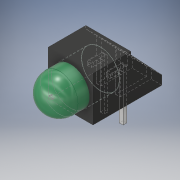
# Autodesk Inventor part: L-1503CB 1GD
Saved by Autodesk Inventor 2019.1 (Build 231200000, 200)
## iProperties
Created: 2021-06-01
Part Number: L-1503CB 1GD
Material: Типовые
Document SubType Name: Modeling
Designer: shawn
Density: 1 g/cm^3
Appearance: По умолчанию
Author: shawn
Autodesk Inventor part; units mm, degrees
ref_plane "YZ Plane" through (0, 0, 0) normal (1, 0, 0) x (0, 1, 0)
ref_plane "XZ Plane" through (0, 0, 0) normal (0, 1, 0) x (-1, 0, 0)
sketch "Эскиз1" plane through (0, 0, 0) normal (1, 0, 0) x (0, 1, 0)
  line L0 (0, 0) -> (6, 0)
  line L1 (6, 0) -> (6, -5.0448)
  line L2 (1.2044, -9.2) -> (0, -9.2)
  line L3 (0, -9.2) -> (0, 0)
  line L4 (1.2044, -9.2) -> (5.6, -5.0448)
  line L5 (5.6, -5.0448) -> (6, -5.0448)
  line L6 (11.4478, 9.2277) -> (11.4478, -15.7017) construction
  line L7 (11.4478, -15.7017) -> (-10.569, -15.7017) construction
  line L8 (-10.569, -15.7017) -> (-10.569, 9.2277) construction
  line L9 (-10.569, 9.2277) -> (11.4478, 9.2277) construction
  dimension "d2" = 0.4
  dimension "d39" = 6
  dimension "d40" = 9.2
  constraints: 13 end point, 2 parallel, 2 perpendicular, 1 horizontal, 3 other
  measures "d2" distance of L1.end L4.end
  measures "d39" distance of L0.start L0.end
  measures "d40" distance of L2.end L0.start
extrude "Выдавливание1" add sketch "Эскиз1" along normal mid plane 6
sketch "Эскиз2" plane through (-3, 0, 0) normal (0, 0, 1) x (1, 0, 0)
  line L0 (6, 6) -> (6, 0) construction
  line L1 (0, 0) -> (6, 6) construction
  line L2 (0, 0) -> (6, 0) construction
  line L3 (6, 0) -> (0, 6) construction
  line L4 (6, 6) -> (0, 6) construction
  circle A0 centre (3, 3) radius 2.55
  point P0 (3, 0)
  dimension "d43" = 5.1
  constraints: 5 end point, 1 centre point, 1 midpoint, 1 perpendicular
  measures "d43" diameter of A0
extrude "Выдавливание2" cut sketch "Эскиз2" against normal blind 4
sketch "Эскиз3" plane through (-3, 0, -9.2) normal (0, -1, 0) x (1, 0, 0)
  line L0 (6, 4.1552) -> (0, 4.1552) construction
  line L1 (6, 0) -> (0, 0) projected
  line L2 (4.57, 4.1552) -> (3.97, 4.1552)
  line L3 (3.97, 4.1552) -> (3.97, 0)
  line L4 (3.97, 0) -> (4.57, 0)
  line L5 (4.57, 0) -> (4.57, 4.1552)
  line L6 (6, 4.1552) -> (0, 4.1552) construction
  line L7 (3, 4.1552) -> (3, 0) construction
  line L8 (1.43, 4.1552) -> (2.03, 4.1552)
  line L9 (2.03, 4.1552) -> (2.03, 0)
  line L10 (2.03, 0) -> (1.43, 0)
  line L11 (1.43, 0) -> (1.43, 4.1552)
  point P0 (3, 9.2)
  point P1 (4.27, 0)
  point P2 (1.73, 0)
  dimension "d46" = 2.54
  dimension "d47" = 0.6
  constraints: 18 end point, 4 midpoint, 4 symmetric about line, 2 parallel, 2 point on line, 1 horizontal, 1 perpendicular
  measures "d46" distance of point (1.73, 0) point (4.27, 0)
  measures "d47" distance of L3.end L4.end
extrude "Выдавливание3" cut sketch "Эскиз3" against normal through all
sketch "Эскиз5" plane through (3, 6, -5.0448) normal (0, 0, -1) x (-1, 0, 0)
  line L0 (1.43, -4.7956) -> (1.43, -0.4) projected
  line L1 (2.03, -0.4) -> (2.03, -4.7956) projected
  line L2 (1.43, -2.7) -> (2.03, -2.7)
  line L3 (2.03, -2.7) -> (2.03, -3.3)
  line L4 (2.03, -3.3) -> (1.43, -3.3)
  line L5 (1.43, -3.3) -> (1.43, -2.7)
  line L6 (2.03, -6) -> (3.97, -6) construction
  line L7 (0, 0) -> (6, 0) construction
  line L8 (1.73, 0) -> (1.73, -6) construction
  line L9 (1.43, -3.3) -> (2.03, -2.7) construction
  line L10 (2.03, -6) -> (1.43, -6) construction
  line L11 (3, 0) -> (3, -6) construction
  line L12 (4.57, -2.7) -> (3.97, -2.7)
  line L13 (3.97, -2.7) -> (3.97, -3.3)
  line L14 (3.97, -3.3) -> (4.57, -3.3)
  line L15 (4.57, -3.3) -> (4.57, -2.7)
  line L16 (4.57, -3.3) -> (3.97, -2.7) construction
  point P0 (1.73, -3)
  point P1 (1.73, -3)
  point P2 (4.27, -3)
  point P3 (4.27, -3)
  dimension "d50" = 0.6
  constraints: 24 end point, 6 midpoint, 6 symmetric about line, 3 point on line, 3 vertical, 2 parallel, 1 horizontal, 1 perpendicular
  measures "d50" distance between parallel lines of L4 L2
extrude "Выдавливание4" cut sketch "Эскиз5" against normal through all
sketch "Эскиз6" plane through (0, 3, -4) normal (0, 0, 1) x (1, 0, 0)
  circle A0 centre (0, 0) radius 2.5
  point P0 (0, -3)
  dimension "d53" = 5
  constraints: 1 centre point
  measures "d53" diameter of A0
extrude "Выдавливание5" add sketch "Эскиз6" along normal blind 8 separate body
fillet "Сопряжение1" radius 2.5 1 edges at (-2.5, 3, 4)
ref_plane "РабПлоскость1" through (1.27, 0, -5.0448) normal (1, 0, 0) x (0, 0, -1)
sketch "Эскиз8" plane through (1.27, 0, -5.0448) normal (1, 0, 0) x (0, 0, -1)
  line L0 (-1.2837, 3.25) -> (0.6552, 3.25)
  line L1 (0.9552, 2.95) -> (0.9552, -3.5)
  line L2 (0.9552, -3.5) -> (0.4552, -3.5)
  line L3 (0.4552, -3.5) -> (0.4552, 2.65)
  line L4 (0.3552, 2.75) -> (-1.2837, 2.75)
  line L5 (-1.2837, 2.75) -> (-1.2837, 3.25)
  line L6 (0, 3.3) -> (-1.0448, 3.3) projected
  line L7 (0, 0) -> (0, 2.7) projected
  line L8 (-5.0448, 0) -> (4.1552, 0) projected
  arc A0 (0.9552, 2.95) -> (0.6552, 3.25) centre (0.6552, 2.95) ccw
  arc A1 (0.4552, 2.65) -> (0.3552, 2.75) centre (0.3552, 2.65) ccw
  line L9 (-5.0448, 6) -> (-5.0448, 0) projected
  point P0 (0.7052, -3.5)
  dimension "d57" = 0.5
  dimension "d58" = 0.05
  dimension "d59" = 0.5
  dimension "d60" = 3.5
  dimension "d61" = 0.3
  dimension "d62" = 0.1
  dimension "d67" = 5.75
  constraints: 12 end point, 5 perpendicular, 4 point on circle, 4 tangent, 2 centre point, 1 horizontal, 1 midpoint
  measures "d57" distance of L4.end L0.start
  measures "d58" distance between parallel lines of L0 L6
  measures "d59" distance of L1.end L2.end
  measures "d60" distance between parallel lines of L2 L8
  measures "d61" radius of A0
  measures "d62" radius of A1
  measures "d67" distance from line of L9 point (0.705, -3.5)
extrude "Выдавливание6" add sketch "Эскиз8" along normal mid plane 0.5 separate body
mirror "Зеркальное отражение1" about plane through (0, 0, 0) normal (1, 0, 0) of "Выдавливание6" bodies 3
sketch "Эскиз9" plane through (-3, 0, 0) normal (0, 0, 1) x (1, 0, 0)
  line L0 (0.4438, 0.8101) -> (0.6148, 0.8101)
  line L1 (0.6148, 0.8101) -> (0.6148, 0.2362)
  line L2 (0.6148, 0.2362) -> (0.4438, 0.2362)
  line L3 (0.4438, 0.2362) -> (0.4438, 0.8101)
  line L4 (0.4438, 0.8101) -> (0.6148, 0.2362) construction
  line L5 (0.6148, 0.8101) -> (0.4438, 0.2362) construction
  line L6 (0.2423, 0.4376) -> (0.8162, 0.4376)
  line L7 (0.8162, 0.4376) -> (0.8162, 0.6086)
  line L8 (0.8162, 0.6086) -> (0.2423, 0.6086)
  line L9 (0.2423, 0.6086) -> (0.2423, 0.4376)
  line L10 (0.2423, 0.4376) -> (0.8162, 0.6086) construction
  line L11 (0.8162, 0.4376) -> (0.2423, 0.6086) construction
  point P0 (3, 0)
  point P1 (0.5293, 0.5231)
  constraints: 24 end point, 4 midpoint, 4 parallel, 4 perpendicular, 2 horizontal
extrude "Выдавливание7" add sketch "Эскиз9" along normal blind 0.1 bodies 1
